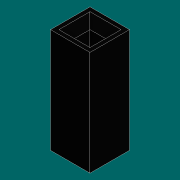
# Autodesk Inventor part: pinShroud
Saved by Autodesk Inventor 2016 SP1 (Build 200210100, 210)
## iProperties
Created: 2016-04-06
Part Number: pinShroud
Material: ABS Plastic
Document SubType Name: Modeling
Designer: sawai
Density: 1.06 g/cm^3
Appearance: Smooth - Black
Author: sawai
Autodesk Inventor part; units mm, degrees
ref_plane "YZ Plane" through (0, 0, 0) normal (1, 0, 0) x (0, 1, 0)
ref_plane "XZ Plane" through (0, 0, 0) normal (0, 1, 0) x (-1, 0, 0)
ref_plane "XY Plane" through (0, 0, 0) normal (0, 0, 1) x (1, 0, 0)
sketch "Sketch1" plane through (0, 0, 0) normal (0, 1, 0) x (-1, 0, 0)
  line L0 (1.27, 1.27) -> (-1.27, 1.27)
  line L1 (-1.27, 1.27) -> (-1.27, -1.27)
  line L2 (-1.27, -1.27) -> (1.27, -1.27)
  line L3 (1.27, -1.27) -> (1.27, 1.27)
  line L4 (1.27, 1.27) -> (-1.27, -1.27) construction
  line L5 (-1.27, 1.27) -> (1.27, -1.27) construction
  line L6 (0.5, 0.5) -> (-0.5, 0.5)
  line L7 (-0.5, 0.5) -> (-0.5, -0.5)
  line L8 (-0.5, -0.5) -> (0.5, -0.5)
  line L9 (0.5, -0.5) -> (0.5, 0.5)
  line L10 (0.5, 0.5) -> (-0.5, -0.5) construction
  line L11 (-0.5, 0.5) -> (0.5, -0.5) construction
  point P0 (0, 0)
  dimension "d0" = 2.54
  dimension "d1" = 2.54
  dimension "d2" = 1
  dimension "d3" = 1
  constraints: 24 end point, 4 midpoint, 4 parallel, 2 horizontal, 2 perpendicular
  measures "d0" distance of L2.end L1.end
  measures "d1" distance of L1.end L0.end
  measures "d2" distance of L8.end L7.end
  measures "d3" distance of L7.end L6.end
extrude "Extrusion1" add sketch "Sketch1" along normal blind 6.73
chamfer "Chamfer1" distance 0.5 angle 45 4 edges at (-0.5, 6.73, 0) (0, 6.73, -0.5) (0.5, 6.73, 0) (0, 6.73, 0.5)
body "Solid1"
